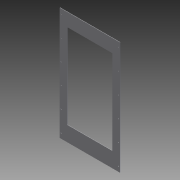
# Autodesk Inventor part: front cover
Saved by Autodesk Inventor 2012 (Build 160160000, 160)
## iProperties
Created: 2012-04-20
Part Number: front cover
Material: Default
Document SubType Name: Modeling
Designer: Puzzles
Density: 1 g/cm^3
Author: Puzzles
Autodesk Inventor part; units mm, degrees
ref_plane "YZ Plane" through (0, 0, 0) normal (1, 0, 0) x (0, 1, 0)
ref_plane "XZ Plane" through (0, 0, 0) normal (0, 1, 0) x (-1, 0, 0)
ref_plane "XY Plane" through (0, 0, 0) normal (0, 0, 1) x (1, 0, 0)
sketch "Sketch1" plane through (0, 0, 0) normal (0, 0, 1) x (1, 0, 0)
  line L0 (-203.2, 381) -> (203.2, 381)
  line L1 (203.2, 381) -> (203.2, -381)
  line L2 (203.2, -381) -> (-203.2, -381)
  line L3 (-203.2, -381) -> (-203.2, 381)
  point P0 (0, 0)
  point P1 (203.2, 0)
  point P2 (0, 381)
  dimension "d0" = 406.4
  dimension "d1" = 762
  constraints: 8 end point, 2 midpoint, 2 parallel, 1 horizontal, 1 horizontal alignment, 1 perpendicular, 1 vertical alignment
  measures "d0" distance of L0.start L0.end
  measures "d1" distance of L0.end L1.end
extrude "Extrusion1" add sketch "Sketch1" along normal blind 3
sketch "Sketch2" plane through (0, 0, 3) normal (0, 0, 1) x (1, 0, 0)
  line L0 (203.2, 381) -> (203.2, -381) projected
  line L1 (-203.2, -381) -> (-203.2, 381) projected
  line L2 (203.2, -381) -> (-203.2, -381) projected
  line L3 (-152.4, 292.1) -> (152.4, 292.1)
  line L4 (152.4, 292.1) -> (152.4, -279.4)
  line L5 (152.4, -279.4) -> (-152.4, -279.4)
  line L6 (-152.4, -279.4) -> (-152.4, 292.1)
  point P0 (0, 0)
  dimension "d4" = 101.6
  dimension "d5" = 50.8
  dimension "d6" = 571.5
  dimension "d7" = 50.8
  constraints: 8 end point, 2 parallel, 1 horizontal, 1 perpendicular
  measures "d4" distance between parallel lines of L2 L5
  measures "d5" distance between parallel lines of L1 L6
  measures "d6" distance of L3.end L4.end
  measures "d7" distance between parallel lines of L0 L4
extrude "Extrusion2" cut sketch "Sketch2" against normal blind 3
sketch "Sketch3" plane through (0, 0, 3) normal (0, 0, 1) x (1, 0, 0)
  line L0 (-203.2, 381) -> (203.2, 381) projected
  line L1 (-203.2, -381) -> (-203.2, 381) projected
  line L2 (203.2, -381) -> (-203.2, -381) projected
  line L3 (0, 473.1075) -> (0, -607.181)
  point P0 (0, 0)
  point P1 (-193.675, 349.25)
  point P2 (-193.675, 209.55)
  point P3 (-193.675, 69.85)
  point P4 (-193.675, -69.85)
  point P5 (-193.675, -209.55)
  point P6 (-193.675, -349.25)
  point P7 (193.675, 349.25)
  point P8 (193.675, 209.55)
  point P9 (193.675, 69.85)
  point P10 (193.675, -69.85)
  point P11 (193.675, -209.55)
  point P12 (193.675, -349.25)
  dimension "d10" = 31.75
  dimension "d11" = 9.525
  dimension "d25" = 139.7
  dimension "d26" = 139.7
  dimension "d27" = 139.7
  dimension "d28" = 139.7
  dimension "d29" = 139.7
  constraints: 6 symmetric about line, 2 end point, 1 perpendicular
  measures "d10" distance from line of L0 point (-193.675, 349.25)
  measures "d11" distance from line of L1 point (-193.675, 349.25)
  measures "d25" distance of point (-193.675, 349.25) point (-193.675, 209.55)
  measures "d26" distance of point (-193.675, 69.85) point (-193.675, 209.55)
  measures "d27" distance of point (-193.675, -69.85) point (-193.675, 69.85)
  measures "d28" distance of point (-193.675, -209.55) point (-193.675, -69.85)
  measures "d29" distance of point (-193.675, -209.55) point (-193.675, -349.25)
hole "Hole2" at (-193.675, 349.25, 3) at (-193.675, 209.55, 3) at (-193.675, 69.85, 3) at (-193.675, -69.85, 3) at (-193.675, -209.55, 3) at (-193.675, -349.25, 3) at (193.675, 349.25, 3) at (193.675, 209.55, 3) at (193.675, 69.85, 3) at (193.675, -69.85, 3) at (193.675, -209.55, 3) at (193.675, -349.25, 3) direction (0, 0, -1) diameter 6.35 end through all
body "Solid1"
